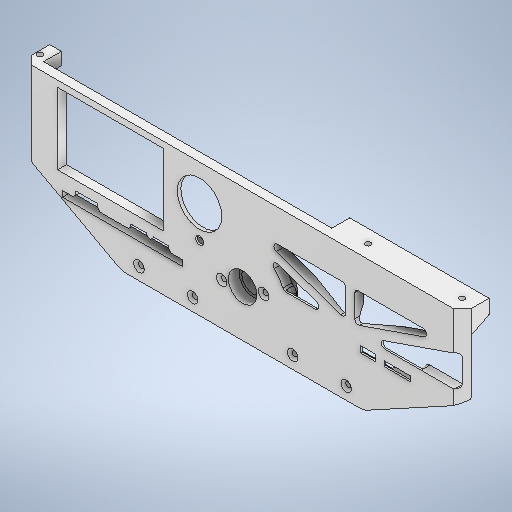
# Autodesk Inventor part: FrontPanel
Saved by Autodesk Inventor 2026.2 (Build 302298000, 298)
## iProperties
Created: 2026-03-31
Part Number: FrontPanel
Material: ABS Plastic
Document SubType Name: Modeling
Designer: gaoet
Density: 1.06 g/cm^3
Appearance: Smooth - White
Author: gaoet
Autodesk Inventor part; units mm, degrees
(part 1 of 2)
ref_plane "YZ Plane" through (0, 0, 0) normal (1, 0, 0) x (0, 1, 0)
ref_plane "XZ Plane" through (0, 0, 0) normal (0, 1, 0) x (-1, 0, 0)
ref_plane "XY Plane" through (0, 0, 0) normal (0, 0, 1) x (1, 0, 0)
sketch "Sketch1" plane through (0, 0, 0) normal (0, 0, 1) x (1, 0, 0)
  line L0 (-125.5, -36.5) -> (125.5, -36.5)
  line L1 (125.5, -36.5) -> (125.5, 36.5)
  line L2 (125.5, 36.5) -> (-125.5, 36.5)
  line L3 (-125.5, 36.5) -> (-125.5, -36.5)
  line L4 (-125.5, -36.5) -> (125.5, 36.5) construction
  line L5 (125.5, -36.5) -> (-125.5, 36.5) construction
  point P0 (0, 0)
  dimension "d0" = 251
  dimension "d1" = 73
  constraints: 12 end point, 2 midpoint, 2 parallel, 1 horizontal, 1 perpendicular
  measures "d0" distance of L2.end L1.end
  measures "d1" distance of L1.end L0.end
extrude "Extrusion1" add sketch "Sketch1" along normal blind 5
sketch "Sketch2" plane through (0, 0, 5) normal (0, 0, 1) x (1, 0, 0)
  line L0 (125.5, -36.5) -> (125.5, 36.5) projected
  line L1 (125.5, 36.5) -> (-125.5, 36.5) projected
  line L2 (-125.5, 36.5) -> (-125.5, -36.5) projected
  line L3 (-125.5, -36.5) -> (125.5, -36.5) projected
  line L4 (-125.5, -6.5) -> (-70.5, -36.5)
  line L5 (125.5, -6.5) -> (70.5, -36.5)
  point P0 (0, 0)
  dimension "d4" = 30
  dimension "d5" = 55
  constraints: 4 end point, 4 point on line, 1 equal length, 1 horizontal alignment
  measures "d4" distance of L2.end L4.start
  measures "d5" distance of L2.end L4.end
extrude "Extrusion2" cut sketch "Sketch2" against normal blind 5 contours L3 L5 L0 | L3 L2 L4
sketch "Sketch3" plane through (0, 0, 5) normal (0, 0, 1) x (1, 0, 0)
  line L0 (-125.5, -6.5) -> (-70.5, -36.5) projected
  line L1 (-70.5, -36.5) -> (70.5, -36.5) projected
  line L2 (70.5, -36.5) -> (125.5, -6.5) projected
  line L3 (125.5, -6.5) -> (125.5, 36.5) projected
  line L4 (125.5, 36.5) -> (-125.5, 36.5) projected
  line L5 (-125.5, 36.5) -> (-125.5, -6.5) projected
  circle A0 centre (0, -12) radius 4.5
  point P0 (0, 0)
  point P1 (0, -36.5)
  dimension "d8" = 9
  dimension "d9" = 24.5
  constraints: 1 centre point, 1 midpoint, 1 vertical alignment
  measures "d8" diameter of A0
  measures "d9" distance of point (0, -36.5) A0.centre
extrude "Extrusion3" cut sketch "Sketch3" against normal through all contours A0
sketch "Sketch4" plane through (0, 0, 0) normal (0, 0, -1) x (-1, 0, 0)
  circle A0 centre (0, -12) radius 4.5 projected
  line L0 (70.5, -36.5) -> (125.5, -6.5) projected
  line L1 (125.5, 36.5) -> (125.5, -6.5) projected
  line L2 (-125.5, 36.5) -> (125.5, 36.5) projected
  line L3 (-125.5, -6.5) -> (-125.5, 36.5) projected
  line L4 (-125.5, -6.5) -> (-70.5, -36.5) projected
  line L5 (70.5, -36.5) -> (-70.5, -36.5) projected
  circle A1 centre (0, -12) radius 8
  circle A2 centre (0, -12) radius 20
  point P0 (0, 0)
  dimension "d12" = 16
  dimension "d13" = 12
  constraints: 2 centre point, 1 coincident
  measures "d12" diameter of A1
  measures "d13" radial gap between concentric circles of A1 A2
extrude "Extrusion4" add sketch "Sketch4" along normal blind 6 contours A2
sketch "Sketch5" plane through (0, -12, 0) normal (0, 0, -1) x (-1, 0, 0)
  circle A0 centre (0, 0) radius 8 projected
  circle A1 centre (0, 0) radius 4.5 projected
  circle A2 centre (0, 0) radius 7
  point P0 (0, 12)
  dimension "d16" = 1
  constraints: 1 centre point
  measures "d16" radial gap between concentric circles of A0 A2
extrude "Extrusion5" add sketch "Sketch5" along normal blind 1 contours A0
fillet "Fillet1" radius 10 2 edges at (-125.5, -6.5, 2.5) (125.5, -6.5, 2.5)
sketch "Sketch11" plane through (0, -12, 0) normal (0, 0, -1) x (-1, 0, 0)
  circle A0 centre (0, 0) radius 7 projected
  circle A1 centre (0, 0) radius 4.5 projected
  circle A2 centre (0, 0) radius 8 projected
  circle A3 centre (0, 0) radius 7 projected
  point P0 (0, 12)
extrude "Extrusion10" cut sketch "Sketch11" along normal through all both and the other way through all contours A0 | A2
sketch "Sketch12" plane through (0, -12, -6) normal (0, 0, -1) x (-1, 0, 0)
  circle A0 centre (0, 0) radius 20 projected
  circle A1 centre (0, 0) radius 8 projected
  circle A2 centre (0, 0) radius 6.5
  point P0 (0, 12)
  dimension "d78" = 1.5
  constraints: 1 centre point, 1 coincident
  measures "d78" radial gap between concentric circles of A1 A2
extrude "Extrusion11" add sketch "Sketch12" against normal blind 5 contours A1
sketch "Sketch14" plane through (0, 0, 0) normal (0, 0, -1) x (-1, 0, 0)
  line L0 (14.15, -7.5) -> (107.15, -7.5) construction
  line L1 (107.15, -7.5) -> (107.15, 33.5) construction
  line L2 (107.15, 33.5) -> (14.15, 33.5) construction
  line L3 (14.15, 33.5) -> (14.15, -7.5) construction
  line L4 (14.15, -7.5) -> (107.15, 33.5) construction
  line L5 (107.15, -7.5) -> (14.15, 33.5) construction
  line L6 (44.85, -6.5) -> (103.15, -6.5)
  line L7 (103.15, -6.5) -> (103.15, 32.5)
  line L8 (103.15, 32.5) -> (44.85, 32.5)
  line L9 (44.85, 32.5) -> (44.85, -6.5)
  line L10 (44.85, -6.5) -> (103.15, 32.5) construction
  line L11 (103.15, -6.5) -> (44.85, 32.5) construction
  line L12 (44.35, 33) -> (103.65, 33)
  line L13 (103.65, 33) -> (103.65, -7)
  line L14 (103.65, -7) -> (44.35, -7)
  line L15 (44.35, -7) -> (44.35, 33)
  line L16 (11.15, -10.5) -> (116.14, -10.5)
  line L17 (116.14, -10.5) -> (116.14, 36.5)
  line L18 (116.14, 36.5) -> (11.15, 36.5)
  line L19 (11.15, 36.5) -> (11.15, -10.5)
  line L20 (11.15, -10.5) -> (116.14, 36.5) construction
  line L21 (116.14, -10.5) -> (11.15, 36.5) construction
  line L22 (44.35, 33) -> (11.15, 33)
  line L23 (44.35, -7) -> (11.15, -7)
  circle A0 centre (24.1039, 16.2969) radius 12.5
  line L24 (11.15, 31) -> (44.35, 31)
  line L25 (11.15, -5) -> (44.35, -5)
  circle A1 centre (24.095, -1.5) radius 2.25
  point P0 (0, 0)
  point P1 (60.65, 13)
  point P2 (74, 13)
  point P3 (63.645, 13)
  dimension "d91" = 93
  dimension "d92" = 41
  dimension "d93" = 58.3
  dimension "d94" = 39
  dimension "d95" = 4
  dimension "d97" = 13
  dimension "d105" = 0.5
  dimension "d108" = 104.99
  dimension "d109" = 47
  dimension "d110" = 3
  dimension "d114" = 25
  dimension "d115" = 12.9539
  dimension "d116" = 20.2031
  dimension "d117" = 2
  dimension "d118" = 2
  dimension "d132" = 4.5
  dimension "d133" = 12.945
  dimension "d134" = 9
  dimension "d169" = 74
  constraints: 52 end point, 9 parallel, 6 horizontal, 6 midpoint, 6 point on line, 4 perpendicular, 2 centre point, 2 horizontal alignment, 3 other
  measures "d91" distance of L2.end L1.end
  measures "d92" distance of L1.end L0.end
  measures "d93" distance of L8.end L7.end
  measures "d94" distance of L6.end L7.end
  measures "d95" distance between parallel lines of L1 L7
  measures "d97" vertical distance of point (0, 0) point (74, 13)
  measures "d105" distance between parallel lines of L8 L12
  measures "d108" distance of L18.end L17.end
  measures "d109" distance of L17.end L16.end
  measures "d110" distance between parallel lines of L19 L3
  measures "d114" diameter of A0
  measures "d115" distance from line of L19 A0.centre
  measures "d116" distance from line of L18 A0.centre
  measures "d117" distance between parallel lines of L22 L24
  measures "d118" distance between parallel lines of L23 L25
  measures "d132" diameter of A1
  measures "d133" distance from line of L19 A1.centre
  measures "d134" distance from line of L16 A1.centre
  measures "d169" horizontal distance of point (0, 0) point (74, 13)
hole "Hole4" at (-107.15, 33.5, 0) at (-107.15, -7.5, 0) at (-14.15, 33.5, 0) at (-14.15, -7.5, 0) direction (0, 0, 1) diameter 3 depth 4
extrude "Extrusion12" cut sketch "Sketch14" against normal through all contours L9 L8 L7 L6 | L12 L13 L14 L15
extrude "Extrusion13" cut sketch "Sketch14" along normal blind 10 contours L9 L8 L7 L6 | L22 L19 L18 L17 L16 L23 L14 L13 L12 | L12 L13 L14 L15 | L15 L24 L19 L22 | L15 L25 L19 L24 | L15 L23 L19 L25 | A0 | A1
extrude "Extrusion14" cut sketch "Sketch14" against normal blind 3 contours L15 L25 L19 L24 | A0 | A1
extrude "Extrusion15" cut sketch "Sketch14" against normal through all contours A0 | A1
sketch "Sketch15" plane through (0, 0, 5) normal (0, 0, 1) x (1, 0, 0)
  circle A0 centre (0, -12) radius 8 projected
  line L0 (-11.7378, -14.4949) -> (0, -12)
  line L1 (0, -12) -> (11.7378, -9.5051)
  line L2 (0, -12) -> (0, 0)
  dimension "d123" = 12
  dimension "d124" = 102
  constraints: 6 end point, 2 collinear, 1 vertical
  measures "d123" distance of L0.start L0.end
  measures "d124" angle of L2 L0
hole "Hole5" at (-11.7378, -14.4949, 5) at (11.7378, -9.5051, 5) direction (0, 0, -1) diameter 3 depth 109 countersink diameter 6 countersink angle 100
sketch "Sketch18" plane through (0, 0, 5) normal (0, 0, 1) x (1, 0, 0)
  line L0 (-70.5, -36.5) -> (70.5, -36.5) projected
  point P0 (0, 0)
  point P1 (-58, -31)
  point P2 (-28, -31)
  point P3 (28, -31)
  point P4 (58, -31)
  point P5 (-67.9501, -36.5)
  point P6 (67.9501, -36.5)
  dimension "d157" = 5.5
  dimension "d158" = 28
  dimension "d159" = 30
  dimension "d160" = 28
  dimension "d161" = 30
  constraints: 3 horizontal alignment
  measures "d157" distance from line of L0 point (-28, -31)
  measures "d158" horizontal distance of point (0, 0) point (-28, -31)
  measures "d159" distance of point (-28, -31) point (-58, -31)
  measures "d160" horizontal distance of point (0, 0) point (28, -31)
  measures "d161" distance of point (58, -31) point (28, -31)
hole "Hole7" at (-58, -31, 5) at (-28, -31, 5) at (28, -31, 5) at (58, -31, 5) direction (0, 0, -1) diameter 3 depth 15 countersink diameter 6 countersink angle 100
sketch "Sketch19" plane through (0, 0, 0) normal (0, 0, -1) x (-1, 0, 0)
  circle A0 centre (-58, -31) radius 1.5 projected
  circle A1 centre (-28, -31) radius 1.5 projected
  circle A2 centre (28, -31) radius 1.5 projected
  circle A3 centre (58, -31) radius 1.5 projected
  line L0 (-125.5, 36.5) -> (125.5, 36.5) projected
  line L1 (-125.5, -0.5637) -> (-125.5, 36.5) projected
  arc A4 (-125.5, -0.5637) -> (-120.2885, -9.3426) centre (-115.5, -0.5637) ccw projected
  line L2 (-120.2885, -9.3426) -> (-70.5, -36.5) projected
  line L3 (70.5, -36.5) -> (-70.5, -36.5) projected
  line L4 (70.5, -36.5) -> (120.2885, -9.3426) projected
  arc A5 (120.2885, -9.3426) -> (125.5, -0.5637) centre (115.5, -0.5637) ccw projected
  line L5 (125.5, 36.5) -> (125.5, -0.5637) projected
  circle A6 centre (107.15, 33.5) radius 1.5 projected
  circle A7 centre (107.15, -7.5) radius 1.5 projected
  circle A8 centre (14.15, 33.5) radius 1.5 projected
  line L6 (11.15, 4.6035) -> (11.15, 31) projected
  line L7 (11.15, 31) -> (44.35, 31) projected
  line L8 (44.35, 31) -> (44.35, 33) projected
  line L9 (44.35, 33) -> (103.65, 33) projected
  line L10 (103.65, 33) -> (103.65, -7) projected
  line L11 (103.65, -7) -> (44.35, -7) projected
  line L12 (44.35, -7) -> (44.35, -5) projected
  line L13 (44.35, -5) -> (11.15, -5) projected
  line L14 (11.15, -5) -> (11.15, -10.5) projected
  line L15 (11.15, -10.5) -> (19.9437, -10.5) projected
  arc A9 (11.15, 4.6035) -> (19.9437, -10.5) centre (0, -12) ccw projected
  circle A10 centre (14.15, -7.5) radius 1.5 projected
  line L16 (116.5, 36.5) -> (116.5, 28.5)
  line L17 (116.5, 28.5) -> (125.5, 28.5)
  line L18 (-125.5, 28.5) -> (0, 28.5)
  line L19 (0, 28.5) -> (0, 36.5)
  line L20 (-45, 36.5) -> (-45, 28.5)
  point P0 (0, 0)
  point P1 (0, 32.5)
  point P2 (-45, 32.5)
  dimension "d170" = 8
  dimension "d171" = 9
  dimension "d261" = 45
  constraints: 10 end point, 5 point on line, 3 midpoint, 3 vertical, 2 perpendicular, 1 horizontal, 1 horizontal alignment
  measures "d170" distance of L16.start L16.end
  measures "d171" distance of L16.end L17.end
  measures "d261" distance of point (0, 32.5) point (-45, 32.5)
extrude "Extrusion17" add sketch "Sketch19" along normal blind 10 contours L0 L20 L18 L1 | L0 L5 L17 L16
chamfer "Chamfer5" distance 5 distance2 10 1 edges at (85.25, 28.5, 0) measured on face at (85.25, 28, 0)
sketch "Sketch20" plane through (-125.5, 36.5, 5) normal (0, 1, 0) x (1, 0, 0)
  line L0 (170.5, 15) -> (251, 15) projected
  line L1 (251, 0) -> (0, 0) projected
  line L2 (9, 5) -> (9, 15) projected
  line L3 (0, 15) -> (0, 0) projected
  line L4 (251, 15) -> (251, 0) projected
  point P0 (4.5, 7.5)
  point P1 (188.25, 7.5)
  point P2 (241, 7.5)
  dimension "d177" = 15
  dimension "d178" = 7.5
  dimension "d179" = 9
  dimension "d180" = 4.5
  dimension "d181" = 10
  dimension "d184" = 52.75
  constraints: 2 horizontal alignment
  measures "d177" distance between parallel lines of L0 L1
  measures "d178" distance from line of point (241, 7.5) L1
  measures "d179" distance between parallel lines of L2 L3
  measures "d180" distance from line of L3 point (4.5, 7.5)
  measures "d181" distance from line of L4 point (241, 7.5)
  measures "d184" distance of point (188.25, 7.5) point (241, 7.5)
hole "Hole8" at (-121, 36.5, -2.5) at (62.75, 36.5, -2.5) at (115.5, 36.5, -2.5) direction (0, -1, 0) diameter 3 depth 10
sketch "Sketch21" plane through (0, 0, 5) normal (0, 0, 1) x (1, 0, 0)
  circle A0 centre (58, -31) radius 3 projected
  circle A1 centre (28, -31) radius 3 projected
  circle A2 centre (-28, -31) radius 3 projected
  circle A3 centre (-58, -31) radius 3 projected
  circle A4 centre (11.7378, -9.5051) radius 3 projected
  circle A5 centre (-11.7378, -14.4949) radius 3 projected
  circle A6 centre (-24.1039, 16.2969) radius 12.5 projected
  circle A7 centre (-24.095, -1.5) radius 2.25 projected
  line L0 (-103.65, -7) -> (-103.65, 33) projected
  line L1 (-103.65, 33) -> (-44.35, 33) projected
  line L2 (-44.35, 33) -> (-44.35, -7) projected
  line L3 (-44.35, -7) -> (-103.65, -7) projected
  line L4 (-70.5, -36.5) -> (70.5, -36.5) projected
  line L5 (70.5, -36.5) -> (120.2885, -9.3426) projected
  arc A8 (120.2885, -9.3426) -> (125.5, -0.5637) centre (115.5, -0.5637) ccw projected
  line L6 (125.5, -0.5637) -> (125.5, 36.5) projected
  line L7 (125.5, 36.5) -> (-125.5, 36.5) projected
  line L8 (-125.5, 36.5) -> (-125.5, -0.5637) projected
  arc A9 (-125.5, -0.5637) -> (-120.2885, -9.3426) centre (-115.5, -0.5637) ccw projected
  line L9 (-120.2885, -9.3426) -> (-70.5, -36.5) projected
  line L10 (125.5, 23.5) -> (45, 23.5) projected
  arc A10 (-19.9437, -10.5) -> (-11.15, 4.6035) centre (0, -12) ccw projected
  line L11 (-19.9437, -10.5) -> (-11.15, -10.5) projected
  line L12 (-11.15, -10.5) -> (-19.9437, -10.5) projected
  line L13 (-19.9437, -10.5) -> (-118.1667, -10.5)
  line L14 (-90.6667, -25.5) -> (-14.7564, -25.5)
  line L15 (0, 36.5) -> (0, 23.5) projected
  line L16 (0, 28.5) -> (0, 36.5) projected
  line L17 (0, 23.5) -> (0, 28.5) projected
  line L18 (0, 36.5) -> (0, 23.5) projected
  line L19 (0, 23.5) -> (0, 8)
  line L20 (-90.6667, -25.5) -> (90.6667, -25.5)
  line L21 (117.8943, -4.9531) -> (70.3443, -30.8895)
  arc A11 (67.9501, -31.5) -> (70.3443, -30.8895) centre (67.9501, -26.5) ccw
  line L22 (67.9501, -31.5) -> (-67.9501, -31.5)
  arc A12 (-70.3443, -30.8895) -> (-67.9501, -31.5) centre (-67.9501, -26.5) ccw
  line L23 (-70.3443, -30.8895) -> (-117.8943, -4.9531)
  arc A13 (-120.5, -0.5637) -> (-117.8943, -4.9531) centre (-115.5, -0.5637) ccw
  line L24 (-120.5, -0.5637) -> (-120.5, 31.5)
  line L25 (-120.5, 31.5) -> (120.5, 31.5)
  line L26 (120.5, 31.5) -> (120.5, -0.5637)
  arc A14 (117.8943, -4.9531) -> (120.5, -0.5637) centre (115.5, -0.5637) ccw
  line L27 (5, 23.5) -> (5, 8)
  line L28 (5, 23.5) -> (80.225, -25.5) construction
  line L29 (14.7564, -25.5) -> (120.5, 31.5) construction
  line L30 (-80.225, -25.5) -> (-19.9437, -10.5) construction
  arc A15 (-24.9296, -10.125) -> (-13.9375, 8.7544) centre (0, -12) ccw
  line L31 (9.5804, 23.5) -> (82.7179, -24.1402)
  line L32 (5, 20.5164) -> (77.7321, -26.8598)
  line L33 (20.0251, -25.5) -> (120.0814, 28.4343)
  line L34 (111.2359, 29.3464) -> (24.3956, -17.464)
  line L35 (-83.4685, -23.7308) -> (-30.2969, -10.5)
  line L36 (-69.8718, -25.5) -> (-24.8932, -14.3079)
  line L37 (18.9492, 4.3073) -> (5, 20.5164)
  line L38 (50.5798, -6.1897) -> (115.5, -0.5637) construction
  line L39 (115.5, -0.5637) -> (120.5, -0.1304)
  line L40 (62.405, -2.6556) -> (120.5525, 2.3836)
  line L41 (58.0225, -8.0541) -> (120.0298, -2.6805)
  point P0 (0, 0)
  point P1 (45.6877, -5.9867)
  point P2 (5, 12.4949)
  point P3 (-107.725, -10.5)
  point P4 (-21.0416, -25.5)
  point P5 (50.4593, -9.0948)
  point P6 (21.5454, -24.6805)
  point P7 (21.0416, -25.5)
  point P8 (75.6446, -25.5)
  point P9 (120.5, 23.5)
  point P10 (110.9276, 23.5)
  point P11 (55.4719, -6.3928)
  point P12 (50.7004, -3.2847)
  point P13 (100.39, 23.5)
  point P14 (83.0399, -3.3767)
  point P15 (120.5, 2.379)
  dimension "d192" = 5.5
  dimension "d193" = 5.5
  dimension "d194" = 5
  dimension "d195" = 5
  dimension "d196" = 5
  dimension "d197" = 2.5
  dimension "d198" = 2.5
  dimension "d199" = 2.5
  dimension "d200" = 2.5
  dimension "d201" = 2.5
  dimension "d202" = 2.5
  dimension "d206" = 2.5
  dimension "d207" = 2.5
  constraints: 50 end point, 22 point on line, 17 point on circle, 9 parallel, 5 centre point, 3 horizontal, 1 collinear, 1 midpoint, 1 tangent, 1 vertical, 5 other
  measures "d192" distance from line of L4 A3.centre
  measures "d193" distance from line of L14 A3.centre
  measures "d194" distance between parallel lines of L5 L21
  measures "d195" distance between parallel lines of L19 L27
  measures "d196" radial gap between concentric circles of A10 A15
  measures "d197" distance between parallel lines of L28 L31
  measures "d198" distance between parallel lines of L32 L28
  measures "d199" distance between parallel lines of L29 L34
  measures "d200" distance between parallel lines of L33 L29
  measures "d201" distance between parallel lines of L36 L30
  measures "d202" distance between parallel lines of L30 L35
  measures "d206" distance from line of point (83.04, -3.377) L40
  measures "d207" distance between parallel lines of L38 L41
extrude "Extrusion18" [suppressed]
fillet "Fillet2" [suppressed]
sketch "Sketch22" plane through (0, 0, 3) normal (0, 0, -1) x (-1, 0, 0)
  circle A0 centre (24.1039, 16.2969) radius 12.5 projected
  circle A1 centre (24.095, -1.5) radius 2.25 projected
  line L0 (44.35, 31) -> (44.35, -5) projected
  line L1 (11.15, 31) -> (44.35, 31) projected
  line L2 (11.15, -5) -> (11.15, 31) projected
  line L3 (44.35, -5) -> (11.15, -5) projected
  line L4 (20.44, 2) -> (27.75, 2)
  line L5 (27.75, 2) -> (27.75, -5)
  line L6 (27.75, -5) -> (20.44, -5)
  line L7 (20.44, -5) -> (20.44, 2)
  line L8 (20.44, 2) -> (27.75, -5) construction
  line L9 (27.75, 2) -> (20.44, -5) construction
  point P0 (0, 0)
  constraints: 12 end point, 3 midpoint, 2 parallel, 1 horizontal, 1 perpendicular
extrude "Extrusion19" cut sketch "Sketch22" against normal blind 1 contours L3 L7 L4 L5
sketch "Sketch23" plane through (-125.5, -0.5637, 5) normal (-1, 0, 0) x (0, 0, 1)
  line L0 (0, 0) -> (-5, 0) projected
  line L1 (0, 37.0637) -> (0, 0) projected
  line L2 (-15, 37.0637) -> (0, 37.0637) projected
  line L3 (-15, 29.0637) -> (-15, 37.0637) projected
  line L4 (-5, 29.0637) -> (-15, 29.0637) projected
  line L5 (-5, 29.0637) -> (-5, 0) projected
  line L6 (-5, 29.0637) -> (-5, 30.0637)
  line L7 (-5, 30.0637) -> (-15, 30.0637)
  point P0 (-5, 0.5637)
  dimension "d210" = 1
  constraints: 4 end point, 1 perpendicular, 1 point on line, 1 vertical
  measures "d210" distance between parallel lines of L4 L7
extrude "Extrusion20" cut sketch "Sketch23" against normal blind 10 contours L4 L3 L7 L6
sketch "Sketch24" plane through (0, 0, 5) normal (0, 0, 1) x (1, 0, 0)
  line L0 (-92.8492, -15.89) -> (-81.6492, -15.89)
  line L1 (-81.6492, -15.89) -> (-81.6492, -12.69)
  line L2 (-81.6492, -12.69) -> (-92.8492, -12.69)
  line L3 (-92.8492, -12.69) -> (-92.8492, -15.89)
  line L4 (-92.8492, -15.89) -> (-81.6492, -12.69) construction
  line L5 (-81.6492, -15.89) -> (-92.8492, -12.69) construction
  line L6 (-62.0971, -15.89) -> (-54.5971, -15.89)
  line L7 (-54.5971, -15.89) -> (-54.5971, -13.29)
  line L8 (-54.5971, -13.29) -> (-62.0971, -13.29)
  line L9 (-62.0971, -13.29) -> (-62.0971, -15.89)
  line L10 (-62.0971, -15.89) -> (-54.5971, -13.29) construction
  line L11 (-54.5971, -15.89) -> (-62.0971, -13.29) construction
  line L12 (-49.4971, -15.89) -> (-41.9971, -15.89)
  line L13 (-41.9971, -15.89) -> (-41.9971, -13.29)
  line L14 (-41.9971, -13.29) -> (-49.4971, -13.29)
  line L15 (-49.4971, -13.29) -> (-49.4971, -15.89)
  line L16 (-49.4971, -15.89) -> (-41.9971, -13.29) construction
  line L17 (-41.9971, -15.89) -> (-49.4971, -13.29) construction
  line L18 (-93.3492, -12.19) -> (-81.1492, -12.19)
  line L19 (-81.1492, -12.19) -> (-81.1492, -16.39)
  line L20 (-81.1492, -16.39) -> (-93.3492, -16.39)
  line L21 (-93.3492, -16.39) -> (-93.3492, -12.19)
  line L22 (-62.5971, -12.79) -> (-54.0971, -12.79)
  line L23 (-54.0971, -12.79) -> (-54.0971, -16.39)
  line L24 (-54.0971, -16.39) -> (-62.5971, -16.39)
  line L25 (-62.5971, -16.39) -> (-62.5971, -12.79)
  line L26 (-49.9971, -12.79) -> (-41.4971, -12.79)
  line L27 (-41.4971, -12.79) -> (-41.4971, -16.39)
  line L28 (-41.4971, -16.39) -> (-49.9971, -16.39)
  line L29 (-49.9971, -16.39) -> (-49.9971, -12.79)
  circle A0 centre (0, -12) radius 6.5 projected
  line L30 (-70.5, -36.5) -> (70.5, -36.5) projected
  line L31 (-100.8492, -18.89) -> (-33.4971, -18.89)
  line L32 (-33.4971, -18.89) -> (-33.4971, -16.39)
  line L33 (-33.4971, -16.39) -> (-100.8492, -16.39)
  line L34 (-100.8492, -16.39) -> (-100.8492, -18.89)
  line L35 (-100.8492, -18.89) -> (-33.4971, -16.39) construction
  line L36 (-33.4971, -18.89) -> (-100.8492, -16.39) construction
  line L37 (-54.5971, -14.59) -> (-49.9971, -14.59)
  point P0 (0, 0)
  point P1 (-87.2492, -14.29)
  point P2 (-58.3471, -14.59)
  point P3 (-45.7471, -14.59)
  point P4 (-67.9501, -36.5)
  point P5 (67.9501, -36.5)
  point P6 (-67.1732, -17.64)
  point P7 (-33.4971, -17.64)
  point P8 (-54.0971, -14.59)
  dimension "d213" = 11.2
  dimension "d214" = 3.2
  dimension "d215" = 0.5
  dimension "d216" = 7.5
  dimension "d217" = 2.6
  dimension "d218" = 0.5
  dimension "d219" = 12.6
  dimension "d220" = 28.9021
  dimension "d221" = 45.7471
  dimension "d222" = 20.61
  dimension "d228" = 2.5
  dimension "d229" = 7.5
  dimension "d230" = 8
  constraints: 74 end point, 14 parallel, 11 midpoint, 7 perpendicular, 4 horizontal, 3 equal length, 3 horizontal alignment, 1 collinear, 1 point on line, 9 other
  measures "d213" distance of L1.end L2.end
  measures "d214" distance of L0.end L1.end
  measures "d215" distance between parallel lines of L2 L18
  measures "d216" distance of L7.end L8.end
  measures "d217" distance of L6.end L7.end
  measures "d218" distance between parallel lines of L8 L22
  measures "d219" distance of point (-45.747, -14.59) point (-58.347, -14.59)
  measures "d220" horizontal distance of point (-58.347, -14.59) point (-87.249, -14.29)
  measures "d221" horizontal distance of A0.centre point (-45.747, -14.59)
  measures "d222" distance between parallel lines of L30 L12
  measures "d228" distance of L33.end L31.start
  measures "d229" distance between parallel lines of L21 L34
  measures "d230" distance from line of point (-33.497, -17.64) L27
extrude "Extrusion21" cut sketch "Sketch24" against normal blind 10 contours L3 L2 L1 L0 | L9 L8 L7 L6 | L15 L14 L13 L12 | L18 L19 L20 L21 | L25 L22 L23 L24 | L23 L37 L29 L33 | L29 L26 L27 L28
chamfer "Chamfer6" [suppressed]
sketch "Sketch25" plane through (0, 0, 0) normal (0, 0, -1) x (-1, 0, 0)
  line L0 (100.8492, -18.89) -> (33.4971, -18.89) projected
  line L1 (33.4971, -18.89) -> (100.8492, -16.39) construction
  line L2 (100.8492, -16.39) -> (100.8492, -18.89) projected
  line L3 (33.4971, -16.39) -> (100.8492, -16.39) projected
  line L4 (33.4971, -18.89) -> (33.4971, -16.39) projected
  line L5 (101.5992, -15.64) -> (101.5992, -19.64)
  line L6 (101.5992, -19.64) -> (32.7471, -19.64)
  line L7 (32.7471, -19.64) -> (32.7471, -15.64)
  line L8 (32.7471, -15.64) -> (101.5992, -15.64)
  line L9 (33.4971, -15.64) -> (33.4971, -16.39)
  line L10 (100.8492, -16.39) -> (100.8492, -15.64)
  point P0 (0, 0)
  dimension "d285" = 0.75
  constraints: 12 end point, 2 point on line, 1 parallel, 1 vertical, 3 other
  measures "d285" distance between parallel lines of L3 L8
extrude "Extrusion22" cut sketch "Sketch25" against normal blind 5 contours L0 L4 L3 L2 | L3 L9 L8 L10
sketch "Sketch26" plane through (0, 0, 5) normal (0, 0, 1) x (1, 0, 0)
  line L0 (-41.4971, -12.79) -> (-41.4971, -15.64) projected
  line L1 (-49.9971, -14.59) -> (-49.9971, -12.79) projected
  line L2 (-49.9971, -12.79) -> (-41.4971, -12.79) projected
  line L3 (-54.0971, -12.79) -> (-54.0971, -14.59) projected
  line L4 (-62.5971, -15.64) -> (-62.5971, -12.79) projected
  line L5 (-62.5971, -12.79) -> (-54.0971, -12.79) projected
  line L6 (-81.1492, -12.19) -> (-81.1492, -15.64) projected
  line L7 (-93.3492, -15.64) -> (-93.3492, -12.19) projected
  line L8 (-93.3492, -12.19) -> (-81.1492, -12.19) projected
  circle A0 centre (58, -31) radius 3 projected
  circle A1 centre (28, -31) radius 3 projected
  circle A2 centre (-28, -31) radius 3 projected
  circle A3 centre (-58, -31) radius 3 projected
  circle A4 centre (11.7378, -9.5051) radius 3 projected
  circle A5 centre (-11.7378, -14.4949) radius 3 projected
  circle A6 centre (-24.1039, 16.2969) radius 12.5 projected
  circle A7 centre (-24.095, -1.5) radius 2.25 projected
  line L9 (-103.65, -7) -> (-103.65, 33) projected
  line L10 (-103.65, 33) -> (-44.35, 33) projected
  line L11 (-44.35, 33) -> (-44.35, -7) projected
  line L12 (-44.35, -7) -> (-103.65, -7) projected
  circle A8 centre (0, -12) radius 8 projected
  line L13 (-70.5, -36.5) -> (70.5, -36.5) projected
  line L14 (70.5, -36.5) -> (120.2885, -9.3426) projected
  arc A9 (120.2885, -9.3426) -> (125.5, -0.5637) centre (115.5, -0.5637) ccw projected
  line L15 (125.5, -0.5637) -> (125.5, 36.5) projected
  line L16 (125.5, 36.5) -> (-125.5, 36.5) projected
  line L17 (-125.5, 36.5) -> (-125.5, -0.5637) projected
  arc A10 (-125.5, -0.5637) -> (-120.2885, -9.3426) centre (-115.5, -0.5637) ccw projected
  line L18 (-120.2885, -9.3426) -> (-70.5, -36.5) projected
  line L19 (66.45, -10) -> (73.95, -10)
  line L20 (73.95, -10) -> (73.95, -7.4)
  line L21 (73.95, -7.4) -> (66.45, -7.4)
  line L22 (66.45, -7.4) -> (66.45, -10)
  line L23 (66.45, -10) -> (73.95, -7.4) construction
  line L24 (73.95, -10) -> (66.45, -7.4) construction
  line L25 (79.765, -10) -> (93.635, -10)
  line L26 (93.635, -10) -> (93.635, -8.15)
  line L27 (93.635, -8.15) -> (79.765, -8.15)
  line L28 (79.765, -8.15) -> (79.765, -10)
  line L29 (79.765, -10) -> (93.635, -8.15) construction
  line L30 (93.635, -10) -> (79.765, -8.15) construction
  line L31 (25, -11.5) -> (97, -11.5)
  line L32 (97, -11.5) -> (97, -10)
  line L33 (97, -10) -> (25, -10)
  line L34 (25, -10) -> (25, -11.5)
  line L35 (25, -11.5) -> (97, -10) construction
  line L36 (97, -11.5) -> (25, -10) construction
  line L37 (79.265, -7.65) -> (94.135, -7.65)
  line L38 (94.135, -7.65) -> (94.135, -10.5)
  line L39 (94.135, -10.5) -> (79.265, -10.5)
  line L40 (79.265, -10.5) -> (79.265, -7.65)
  line L41 (-54.5971, -13.29) -> (-62.0971, -13.29) projected
  line L42 (-62.0971, -13.29) -> (-62.0971, -15.89) projected
  line L43 (65.95, -6.9) -> (74.45, -6.9)
  line L44 (74.45, -6.9) -> (74.45, -10.5)
  line L45 (74.45, -10.5) -> (65.95, -10.5)
  line L46 (65.95, -10.5) -> (65.95, -6.9)
  line L47 (65.95, -10.5) -> (74.45, -10.5)
  line L48 (74.45, -10.5) -> (74.45, -11)
  line L49 (74.45, -11) -> (65.95, -11)
  line L50 (65.95, -11) -> (65.95, -10.5)
  line L51 (79.265, -10.5) -> (94.135, -10.5)
  line L52 (94.135, -10.5) -> (94.135, -11)
  line L53 (94.135, -11) -> (79.265, -11)
  line L54 (79.265, -11) -> (79.265, -10.5)
  line L55 (65.95, -7.4) -> (74.45, -7.4)
  line L56 (79.265, -8.15) -> (94.317, -8.15)
  line L57 (-33.4971, -18.89) -> (-100.8492, -18.89) projected
  line L58 (-100.8492, -18.89) -> (-100.8492, -15.64) projected
  line L59 (-41.4971, -15.64) -> (-33.4971, -15.64) projected
  line L60 (-33.4971, -15.64) -> (-33.4971, -18.89) projected
  line L61 (-100.8492, -15.64) -> (-93.3492, -15.64) projected
  line L62 (-81.1492, -15.64) -> (-62.5971, -15.64) projected
  line L63 (-54.0971, -14.59) -> (-49.9971, -14.59) projected
  point P0 (0, 0)
  point P1 (70.2, -8.7)
  point P2 (86.7, -9.075)
  point P3 (61, -10.75)
  point P4 (97, -10.75)
  point P5 (94.135, -8.15)
  dimension "d233" = 25
  dimension "d234" = 1.5
  dimension "d235" = 72
  dimension "d236" = 28.5
  dimension "d237" = 13.87
  dimension "d238" = 1.85
  dimension "d239" = 10.3
  dimension "d240" = 0.5
  dimension "d241" = 16.5
  dimension "d242" = 0.5
  dimension "d247" = 0.5
  constraints: 72 end point, 16 parallel, 7 horizontal, 7 midpoint, 7 perpendicular, 4 collinear, 3 point on line, 2 vertical alignment, 1 horizontal alignment, 6 other
  measures "d233" distance between parallel lines of L13 L31
  measures "d234" distance of L33.end L31.start
  measures "d235" distance of L32.end L33.end
  measures "d236" distance from line of L15 point (97, -10.75)
  measures "d237" distance of L26.end L27.end
  measures "d238" distance of L25.end L26.end
  measures "d239" distance from line of L32 point (86.7, -9.075)
  measures "d240" distance between parallel lines of L27 L37
  measures "d241" horizontal distance of point (86.7, -9.075) point (70.2, -8.7)
  measures "d242" distance between parallel lines of L21 L43
  measures "d247" distance between parallel lines of L53 L39
extrude "Extrusion23" cut sketch "Sketch26" against normal through all contours L22 L21 L20 L19 | L33 L46 L55 L22 | L19 L33 L44 L45 L46 | L20 L55 L44 L33 | L45 L48 L49 L50 | L40 L56 L28 L33 | L33 L25 L38 L39 L40 | L28 L27 L26 L25 | L39 L52 L53 L54 | L26 L56 L38 L33
sketch "Sketch27" plane through (0, 0, 0) normal (0, 0, -1) x (-1, 0, 0)
  line L0 (-25, -11.5) -> (-97, -11.5) projected
  line L1 (-97, -10) -> (-25, -10) projected
  line L2 (-25, -10) -> (-25, -11.5) projected
  line L3 (-97, -11.5) -> (-97, -10) projected
  point P0 (0, 0)
extrude "Extrusion24" cut sketch "Sketch27" against normal blind 4
sketch "Sketch28" plane through (0, 0, 0) normal (0, 0, -1) x (-1, 0, 0)
  line L0 (-97, -10) -> (-94.135, -10) construction
  line L1 (-94.135, -10) -> (-94.135, -8.15) construction
  line L2 (-94.135, -8.15) -> (-79.265, -8.15) construction
  line L3 (-79.265, -8.15) -> (-79.265, -10) construction
  line L4 (-79.265, -10) -> (-74.45, -10) construction
  line L5 (-74.45, -10) -> (-74.45, -7.4) construction
  line L6 (-74.45, -7.4) -> (-65.95, -7.4) construction
  line L7 (-65.95, -7.4) -> (-65.95, -10) construction
  line L8 (-65.95, -10) -> (-25, -10) construction
  line L9 (-25, -10) -> (-25, -11.5) construction
  line L10 (-25, -11.5) -> (-97, -11.5) construction
  line L11 (-97, -11.5) -> (-97, -10) construction
  line L12 (41.4971, -15.64) -> (41.4971, -12.79) construction
  line L13 (41.4971, -12.79) -> (49.9971, -12.79) construction
  line L14 (49.9971, -12.79) -> (49.9971, -14.59) construction
  line L15 (54.0971, -14.59) -> (54.0971, -12.79) construction
  line L16 (54.0971, -12.79) -> (62.5971, -12.79) construction
  line L17 (62.5971, -12.79) -> (62.5971, -15.64) construction
  line L18 (81.1492, -15.64) -> (81.1492, -12.19) construction
  line L19 (81.1492, -12.19) -> (93.3492, -12.19) projected
  line L20 (93.3492, -12.19) -> (93.3492, -15.64) projected
  line L21 (100.8492, -15.64) -> (100.8492, -18.89) projected
  line L22 (100.8492, -18.89) -> (33.4971, -18.89) projected
  line L23 (116.5, 29.5) -> (116.5, 36.5) projected
  line L24 (-45, 36.5) -> (116.5, 36.5) projected
  line L25 (-125.5, 23.5) -> (-45, 23.5) construction
  line L26 (-125.5, -0.5637) -> (-125.5, 23.5) construction
  arc A0 (-125.5, -0.5637) -> (-120.2885, -9.3426) centre (-115.5, -0.5637) ccw construction
  line L27 (-120.2885, -9.3426) -> (-70.5, -36.5) construction
  line L28 (70.5, -36.5) -> (-70.5, -36.5) construction
  line L29 (70.5, -36.5) -> (120.2885, -9.3426) projected
  arc A1 (120.2885, -9.3426) -> (125.5, -0.5637) centre (115.5, -0.5637) ccw projected
  line L30 (125.5, 29.5) -> (125.5, -0.5637) projected
  line L31 (125.5, 29.5) -> (116.5, 29.5) projected
  circle A2 centre (-58, -31) radius 1.5 construction
  circle A3 centre (-28, -31) radius 1.5 construction
  circle A4 centre (28, -31) radius 1.5 construction
  circle A5 centre (58, -31) radius 1.5 construction
  circle A6 centre (107.15, 33.5) radius 1.5 projected
  circle A7 centre (107.15, -7.5) radius 1.5 projected
  circle A8 centre (14.15, 33.5) radius 1.5 construction
  line L32 (11.15, 4.6035) -> (11.15, 31) construction
  line L33 (11.15, 31) -> (44.35, 31) construction
  line L34 (44.35, 31) -> (44.35, 33) construction
  line L35 (44.35, 33) -> (103.65, 33) projected
  line L36 (103.65, 33) -> (103.65, -7) projected
  line L37 (103.65, -7) -> (44.35, -7) projected
  line L38 (44.35, -7) -> (44.35, -5) construction
  line L39 (44.35, -5) -> (11.15, -5) construction
  line L40 (11.15, -5) -> (11.15, -10.5) construction
  line L41 (11.15, -10.5) -> (19.9437, -10.5) construction
  arc A9 (11.15, 4.6035) -> (19.9437, -10.5) centre (0, -12) ccw construction
  circle A10 centre (14.15, -7.5) radius 1.5 construction
  circle A11 centre (-11.7378, -9.5051) radius 1.5 construction
  circle A12 centre (11.7378, -14.4949) radius 1.5 construction
  line L42 (19.9437, -10.5) -> (11.15, -10.5) construction
  line L43 (11.15, -10.5) -> (11.15, 4.6035) construction
  arc A13 (11.15, 4.6035) -> (19.9437, -10.5) centre (0, -12) ccw construction
  circle A14 centre (0, -12) radius 6.5 construction
  line L44 (-19.4638, -7.4) -> (-122.7983, -7.4) construction
  line L45 (5, 18.5) -> (5, 31.5) construction
  line L46 (5, 31.5) -> (111.5, 31.5)
  line L47 (111.5, 31.5) -> (111.5, 24.5)
  line L48 (111.5, 24.5) -> (120.5, 24.5)
  line L49 (120.5, 24.5) -> (120.5, -0.5637)
  arc A15 (117.8943, -4.9531) -> (120.5, -0.5637) centre (115.5, -0.5637) ccw
  line L50 (117.8943, -4.9531) -> (70.3443, -30.8895)
  arc A16 (67.9501, -31.5) -> (70.3443, -30.8895) centre (67.9501, -26.5) ccw construction
  line L51 (67.9501, -31.5) -> (-67.9501, -31.5) construction
  arc A17 (-70.3443, -30.8895) -> (-67.9501, -31.5) centre (-67.9501, -26.5) ccw construction
  line L52 (-70.3443, -30.8895) -> (-117.8943, -4.9531) construction
  arc A18 (-120.5, -0.5637) -> (-117.8943, -4.9531) centre (-115.5, -0.5637) ccw
  line L53 (-120.5, -0.5637) -> (-120.5, 18.5)
  line L54 (-120.5, 18.5) -> (5, 18.5)
  line L55 (-23.0833, -2.4) -> (-120.1506, -2.4)
  circle A19 centre (0, -12) radius 25
  line L56 (0, 18.5) -> (0, 13)
  line L57 (-120.5, 18.5) -> (-60.25, -2.4)
  line L58 (-60.25, -2.4) -> (0, 18.5)
  line L59 (-60.25, 18.5) -> (-60.25, -2.4)
  line L60 (-112.8718, 18.5) -> (-52.6218, -2.4)
  line L61 (-120.5, 15.8539) -> (-67.8782, -2.4)
  line L62 (-62.75, 18.5) -> (-62.75, -2.4)
  line L63 (-57.75, 18.5) -> (-57.75, -2.4)
  line L64 (-67.8782, -2.4) -> (2.5, 22.0134)
  line L65 (2.5, 22.0134) -> (2.5, 13.9659)
  line L66 (-52.6218, -2.4) -> (7.7362, 18.5374)
  line L67 (-13.3981, 11.2062) -> (0, -12)
  line L68 (-45, 36.5) -> (-45, 23.5) projected
  line L69 (33.4971, -15.64) -> (41.4971, -15.64) projected
  line L70 (62.5971, -15.64) -> (81.1492, -15.64) projected
  line L71 (93.3492, -15.64) -> (100.8492, -15.64) projected
  line L72 (33.4971, -18.89) -> (33.4971, -15.64) projected
  line L73 (49.9971, -14.59) -> (54.0971, -14.59) projected
  point P0 (0, 0)
  point P1 (-57.75, 1.1134)
  point P2 (-7.6282, 18.5)
  point P3 (0, 15.8539)
  point P4 (-62.75, 1.1134)
  point P5 (-12.5, 9.6506)
  dimension "d248" = 5
  dimension "d249" = 5
  dimension "d250" = 5
  dimension "d251" = 2.5
  dimension "d252" = 2.5
  dimension "d253" = 2.5
  dimension "d254" = 2.5
  dimension "d255" = 2.5
  dimension "d256" = 2.5
  dimension "d260" = 30
  constraints: 46 end point, 13 point on circle, 6 point on line, 5 centre point, 4 parallel, 2 horizontal, 2 vertical, 1 coincident, 1 collinear, 1 equal length, 1 midpoint, 1 vertical alignment, 19 other
  measures "d248" distance between parallel lines of L25 L54
  measures "d250" radial gap between concentric circles of A9 A19
  measures "d251" distance between parallel lines of L57 L60
  measures "d252" distance between parallel lines of L61 L57
  measures "d253" distance between parallel lines of L59 L62
  measures "d254" distance between parallel lines of L59 L63
  measures "d255" distance between parallel lines of L58 L64
  measures "d256" distance between parallel lines of L58 L66
  measures "d260" angle of L56 L67
extrude "Extrusion25" cut sketch "Sketch28" against normal blind 10 contours L53 L61 L55 A18 | L54 L62 L60 | L66 L67 A19 L55 | L63 L54 L64
fillet "Fillet3" radius 2 13 edges at (67.8782, -2.4, 2.5) (120.5, 15.8539, 2.5) (120.1506, -2.4, 2.5) (112.8718, 18.5, 2.5) (62.75, 1.1134, 2.5) (62.75, 18.5, 2.5) (57.75, 18.5, 2.5) (57.75, 1.1134, 2.5) (52.6218, -2.4, 2.5) (7.6282, 18.5, 2.5) (23.0833, -2.4, 2.5) (13.3981, 11.2062, 2.5) (12.5, 9.6506, 2.5)
sketch "Sketch29" plane through (0, 0, 5) normal (0, 0, 1) x (1, 0, 0)
  line L0 (101.6591, 14.6105) -> (65.4055, 2.0345) projected
  arc A0 (62.75, 3.9241) -> (65.4055, 2.0345) centre (64.75, 3.9241) ccw projected
  line L1 (62.75, 3.9241) -> (62.75, 16.5) projected
  arc A1 (64.75, 18.5) -> (62.75, 16.5) centre (64.75, 16.5) ccw projected
  line L2 (64.75, 18.5) -> (101.0036, 18.5) projected
  arc A2 (101.6591, 14.6105) -> (101.0036, 18.5) centre (101.0036, 16.5) ccw projected
  line L3 (118.5, -2.4) -> (79.7464, -2.4) projected
  arc A3 (79.0909, 1.4895) -> (79.7464, -2.4) centre (79.7464, -0.4) ccw projected
  line L4 (79.0909, 1.4895) -> (117.8445, 14.9327) projected
  arc A4 (120.5, 13.0432) -> (117.8445, 14.9327) centre (118.5, 13.0432) ccw projected
  line L5 (120.5, 13.0432) -> (120.5, -0.4) projected
  arc A5 (118.5, -2.4) -> (120.5, -0.4) centre (118.5, -0.4) ccw projected
  line L6 (57.75, 16.5) -> (57.75, 3.9241) projected
  arc A6 (55.0945, 2.0345) -> (57.75, 3.9241) centre (55.75, 3.9241) ccw projected
  line L7 (55.0945, 2.0345) -> (18.8409, 14.6105) projected
  arc A7 (19.4964, 18.5) -> (18.8409, 14.6105) centre (19.4964, 16.5) ccw projected
  line L8 (19.4964, 18.5) -> (55.75, 18.5) projected
  arc A8 (57.75, 16.5) -> (55.75, 18.5) centre (55.75, 16.5) ccw projected
  line L9 (40.7536, -2.4) -> (24.3811, -2.4) projected
  arc A9 (22.5751, -1.2593) -> (24.3811, -2.4) centre (24.3811, -0.4) ccw projected
  arc A10 (22.5751, -1.2593) -> (17.6459, 5.7093) centre (0, -12) ccw projected
  arc A11 (19.7131, 9.0156) -> (17.6459, 5.7093) centre (19.0576, 7.1261) ccw projected
  line L10 (19.7131, 9.0156) -> (41.4091, 1.4895) projected
  arc A12 (40.7536, -2.4) -> (41.4091, 1.4895) centre (40.7536, -0.4) ccw projected
  line L11 (94.135, -11) -> (79.265, -11) projected
  line L12 (79.265, -11) -> (79.265, -8.15) projected
  line L13 (79.265, -8.15) -> (94.135, -8.15) projected
  line L14 (94.135, -8.15) -> (94.135, -11) projected
  line L15 (74.45, -11) -> (65.95, -11) projected
  line L16 (65.95, -11) -> (65.95, -7.4) projected
  line L17 (65.95, -7.4) -> (74.45, -7.4) projected
  line L18 (74.45, -7.4) -> (74.45, -11) projected
  line L19 (-41.4971, -12.79) -> (-41.4971, -15.64) projected
  line L20 (-49.9971, -14.59) -> (-49.9971, -12.79) projected
  line L21 (-49.9971, -12.79) -> (-41.4971, -12.79) projected
  line L22 (-54.0971, -12.79) -> (-54.0971, -14.59) projected
  line L23 (-62.5971, -15.64) -> (-62.5971, -12.79) projected
  line L24 (-62.5971, -12.79) -> (-54.0971, -12.79) projected
  line L25 (-81.1492, -12.19) -> (-81.1492, -15.64) projected
  line L26 (-93.3492, -15.64) -> (-93.3492, -12.19) projected
  line L27 (-93.3492, -12.19) -> (-81.1492, -12.19) projected
  circle A13 centre (58, -31) radius 3 projected
  circle A14 centre (28, -31) radius 3 projected
  circle A15 centre (-28, -31) radius 3 projected
  circle A16 centre (-58, -31) radius 3 projected
  circle A17 centre (11.7378, -9.5051) radius 3 projected
  circle A18 centre (-11.7378, -14.4949) radius 3 projected
  circle A19 centre (-24.1039, 16.2969) radius 12.5 projected
  circle A20 centre (-24.095, -1.5) radius 2.25 projected
  line L28 (-103.65, -7) -> (-103.65, 33) projected
  line L29 (-103.65, 33) -> (-44.35, 33) projected
  line L30 (-44.35, 33) -> (-44.35, -7) projected
  line L31 (-44.35, -7) -> (-103.65, -7) projected
  circle A21 centre (0, -12) radius 8 projected
  arc A22 (120.2885, -9.3426) -> (125.5, -0.5637) centre (115.5, -0.5637) ccw projected
  line L32 (125.5, -0.5637) -> (125.5, 36.5) projected
  line L33 (125.5, 36.5) -> (-125.5, 36.5) projected
  line L34 (-125.5, 36.5) -> (-125.5, -0.5637) projected
  arc A23 (-125.5, -0.5637) -> (-120.2885, -9.3426) centre (-115.5, -0.5637) ccw projected
  line L35 (-120.2885, -9.3426) -> (-70.5, -36.5) projected
  line L36 (-70.5, -36.5) -> (70.5, -36.5) projected
  line L37 (70.5, -36.5) -> (120.2885, -9.3426) projected
  line L38 (-70.5, -36.5) -> (-67.75, -38)
  line L39 (-67.75, -38) -> (67.75, -38)
  line L40 (67.75, -38) -> (70.5, -36.5)
  line L41 (-33.4971, -18.89) -> (-100.8492, -18.89) projected
  line L42 (-100.8492, -18.89) -> (-100.8492, -15.64) projected
  line L43 (-41.4971, -15.64) -> (-33.4971, -15.64) projected
  line L44 (-33.4971, -15.64) -> (-33.4971, -18.89) projected
  line L45 (-100.8492, -15.64) -> (-93.3492, -15.64) projected
  line L46 (-81.1492, -15.64) -> (-62.5971, -15.64) projected
  line L47 (-54.0971, -14.59) -> (-49.9971, -14.59) projected
  point P0 (0, 0)
  dimension "d262" = 1.5
  constraints: 6 end point, 2 collinear, 1 horizontal
  measures "d262" distance between parallel lines of L36 L39
extrude "Extrusion26" add sketch "Sketch29" against normal up to surface (5 mm away) contours L40 L39 L38 L36
fillet "Fillet4" radius 10 2 edges at (-67.75, -38, 2.5) (67.75, -38, 2.5)
sketch "Sketch30" plane through (0, 0, 5) normal (0, 0, 1) x (1, 0, 0)
  line L0 (101.6591, 14.6105) -> (65.4055, 2.0345) projected
  arc A0 (62.75, 3.9241) -> (65.4055, 2.0345) centre (64.75, 3.9241) ccw projected
  line L1 (62.75, 3.9241) -> (62.75, 16.5) projected
  arc A1 (64.75, 18.5) -> (62.75, 16.5) centre (64.75, 16.5) ccw projected
  line L2 (64.75, 18.5) -> (101.0036, 18.5) projected
  arc A2 (101.6591, 14.6105) -> (101.0036, 18.5) centre (101.0036, 16.5) ccw projected
  line L3 (118.5, -2.4) -> (79.7464, -2.4) projected
  arc A3 (79.0909, 1.4895) -> (79.7464, -2.4) centre (79.7464, -0.4) ccw projected
  line L4 (79.0909, 1.4895) -> (117.8445, 14.9327) projected
  arc A4 (120.5, 13.0432) -> (117.8445, 14.9327) centre (118.5, 13.0432) ccw projected
  line L5 (120.5, 13.0432) -> (120.5, -0.4) projected
  arc A5 (118.5, -2.4) -> (120.5, -0.4) centre (118.5, -0.4) ccw projected
  line L6 (57.75, 16.5) -> (57.75, 3.9241) projected
  arc A6 (55.0945, 2.0345) -> (57.75, 3.9241) centre (55.75, 3.9241) ccw projected
  line L7 (55.0945, 2.0345) -> (18.8409, 14.6105) projected
  arc A7 (19.4964, 18.5) -> (18.8409, 14.6105) centre (19.4964, 16.5) ccw projected
  line L8 (19.4964, 18.5) -> (55.75, 18.5) projected
  arc A8 (57.75, 16.5) -> (55.75, 18.5) centre (55.75, 16.5) ccw projected
  line L9 (40.7536, -2.4) -> (24.3811, -2.4) projected
  arc A9 (22.5751, -1.2593) -> (24.3811, -2.4) centre (24.3811, -0.4) ccw projected
  arc A10 (22.5751, -1.2593) -> (17.6459, 5.7093) centre (0, -12) ccw projected
  arc A11 (19.7131, 9.0156) -> (17.6459, 5.7093) centre (19.0576, 7.1261) ccw projected
  line L10 (19.7131, 9.0156) -> (41.4091, 1.4895) projected
  arc A12 (40.7536, -2.4) -> (41.4091, 1.4895) centre (40.7536, -0.4) ccw projected
  line L11 (94.135, -11) -> (79.265, -11) projected
  line L12 (79.265, -11) -> (79.265, -8.15) projected
  line L13 (79.265, -8.15) -> (94.135, -8.15) projected
  line L14 (94.135, -8.15) -> (94.135, -11) projected
  line L15 (74.45, -11) -> (65.95, -11) projected
  line L16 (65.95, -11) -> (65.95, -7.4) projected
  line L17 (65.95, -7.4) -> (74.45, -7.4) projected
  line L18 (74.45, -7.4) -> (74.45, -11) projected
  line L19 (-41.4971, -12.79) -> (-41.4971, -15.64) projected
  line L20 (-49.9971, -14.59) -> (-49.9971, -12.79) projected
  line L21 (-49.9971, -12.79) -> (-41.4971, -12.79) projected
  line L22 (-54.0971, -12.79) -> (-54.0971, -14.59) projected
  line L23 (-62.5971, -15.64) -> (-62.5971, -12.79) projected
  line L24 (-62.5971, -12.79) -> (-54.0971, -12.79) projected
  line L25 (-81.1492, -12.19) -> (-81.1492, -15.64) projected
  line L26 (-93.3492, -15.64) -> (-93.3492, -12.19) projected
  line L27 (-93.3492, -12.19) -> (-81.1492, -12.19) projected
  circle A13 centre (58, -31) radius 3 projected
  circle A14 centre (28, -31) radius 3 projected
  circle A15 centre (-28, -31) radius 3 projected
  circle A16 centre (-58, -31) radius 3 projected
  circle A17 centre (11.7378, -9.5051) radius 3 projected
  circle A18 centre (-11.7378, -14.4949) radius 3 projected
  circle A19 centre (-24.1039, 16.2969) radius 12.5 projected
  circle A20 centre (-24.095, -1.5) radius 2.25 projected
  line L28 (-103.65, -7) -> (-103.65, 33) projected
  line L29 (-103.65, 33) -> (-44.35, 33) projected
  line L30 (-44.35, 33) -> (-44.35, -7) projected
  line L31 (-44.35, -7) -> (-103.65, -7) projected
  circle A21 centre (0, -12) radius 8 projected
  arc A22 (65.2001, -38) -> (69.9886, -36.779) centre (65.2001, -28) ccw projected
  line L32 (69.9886, -36.779) -> (120.2885, -9.3426) projected
  arc A23 (120.2885, -9.3426) -> (125.5, -0.5637) centre (115.5, -0.5637) ccw projected
  line L33 (125.5, -0.5637) -> (125.5, 36.5) projected
  line L34 (125.5, 36.5) -> (-125.5, 36.5) projected
  line L35 (-125.5, 36.5) -> (-125.5, -0.5637) projected
  arc A24 (-125.5, -0.5637) -> (-120.2885, -9.3426) centre (-115.5, -0.5637) ccw projected
  line L36 (-120.2885, -9.3426) -> (-69.9886, -36.779) projected
  arc A25 (-69.9886, -36.779) -> (-65.2001, -38) centre (-65.2001, -28) ccw projected
  line L37 (-65.2001, -38) -> (65.2001, -38) projected
  line L38 (123, 36.5) -> (123, -7.178)
  line L39 (-123, 36.5) -> (-123, -7.178)
  line L40 (-125.5, 36.5) -> (-125.5, -0.5637) projected
  line L41 (-33.4971, -18.89) -> (-100.8492, -18.89) projected
  line L42 (-100.8492, -18.89) -> (-100.8492, -15.64) projected
  line L43 (-41.4971, -15.64) -> (-33.4971, -15.64) projected
  line L44 (-33.4971, -15.64) -> (-33.4971, -18.89) projected
  line L45 (-100.8492, -15.64) -> (-93.3492, -15.64) projected
  line L46 (-81.1492, -15.64) -> (-62.5971, -15.64) projected
  line L47 (-54.0971, -14.59) -> (-49.9971, -14.59) projected
  point P0 (0, 0)
  dimension "d266" = 2.5
  dimension "d267" = 2.5
  constraints: 4 end point, 2 point on circle, 2 point on line, 2 vertical, 1 other
  measures "d266" distance between parallel lines of L35 L39
  measures "d267" distance between parallel lines of L33 L38
extrude "Extrusion27" cut sketch "Sketch30" against normal through all contours L38 L34 L33 A23 | A24 L35 L34 L39